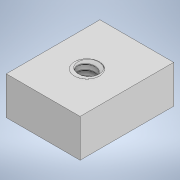
# Autodesk Inventor part: Part1
Saved by Autodesk Inventor 2020.2 (Build 242310000, 310)
## iProperties
Created: 2020-04-14
Part Number: Part1
Material: Generic
Document SubType Name: Modeling
Designer: robst
Density: 1 g/cm^3
Appearance: Default
Author: robst
Autodesk Inventor part; units mm, degrees
ref_plane "YZ Plane" through (0, 0, 0) normal (1, 0, 0) x (0, 1, 0)
ref_plane "XZ Plane" through (0, 0, 0) normal (0, 1, 0) x (-1, 0, 0)
ref_plane "XY Plane" through (0, 0, 0) normal (0, 0, 1) x (1, 0, 0)
sketch "Sketch1" plane through (0, 0, 0) normal (0, 0, 1) x (1, 0, 0)
  line L0 (-11.3242, -3.9027) -> (8.701, -3.9027)
  line L1 (8.701, -3.9027) -> (8.701, 6.3978)
  line L2 (8.701, 6.3978) -> (-11.3242, 6.3978)
  line L3 (-11.3242, 6.3978) -> (-11.3242, -3.9027)
  point P0 (0, 0)
  constraints: 8 end point, 2 parallel, 1 horizontal, 1 perpendicular
extrude "Extrusion1" add sketch "Sketch1" along normal blind 25.4
sketch "Sketch2" plane through (-11.3242, 6.3978, 0) normal (0, 1, 0) x (1, 0, 0)
  point P0 (11.3242, 0)
  point P1 (9.7887, -13.3075)
hole "Hole1" at (-1.5355, 6.3978, 13.3075) direction (0, -1, 0) diameter 6.7564 end through all clearance for "Flat Head Machine Screw (82)" size "1/4" standard "Ansi Unified Screw Threads"
thread "Thread1" size "5/16-18 UNC" class "2B" standard "ANSI Unified Screw Threads" full length
sketch "Sketch4" plane through (-1.5355, 6.3978, 13.3075) normal (1, 0, 0) x (0, 0, 1)
  line L0 (3.3782, 0) -> (3.3782, 10.3005)
  line L1 (3.3782, 10.3005) -> (2.3319, 10.3005)
  line L2 (2.3319, 10.3005) -> (2.3319, 0)
  line L3 (2.3319, 0) -> (3.3782, 0)
  line L4 (0, -3.9066) -> (0, 12.6684) projected
  constraints: 8 end point
revolve "Revolution1" add sketch "Sketch4" angle 360 about axis through (-1.5355, 6.3978, 13.3075) along (0, -1, 0) separate body
sketch "Sketch3" plane through (-1.5355, 6.3978, 16.6857) normal (-1, 0, 0) x (0, -1, 0)
  line L0 (-0.8233, -0.0715) -> (-0.7057, -0.0715) construction
  line L1 (0.1175, -0.9751) -> (-0.0001, -1.201) construction
  line L2 (-1.4112, -1.201) -> (-1.5288, -0.9751) construction
  line L3 (-0.5881, -0.0715) -> (-0.7057, 0.1544) construction
  line L4 (-0.7057, 0.1544) -> (-0.8233, -0.0715) construction
  line L5 (-1.4112, -1.201) -> (-1.2936, -0.9751) construction
  line L6 (-0.5881, -0.0715) -> (-0.1177, -0.9751)
  line L7 (-1.5288, -0.9751) -> (-1.2936, -0.9751) construction
  arc A0 (-1.5288, -0.9751) -> (-1.4112, -1.0465) centre (-1.4112, -0.9139) ccw construction
  line L8 (0.1175, -0.9751) -> (-0.1177, -0.9751) construction
  line L9 (-1.4112, -1.201) -> (-1.4112, -0.9751) construction
  line L10 (-0.0001, -1.201) -> (-0.0001, -0.9751) construction
  line L11 (-0.7057, 0.1544) -> (-0.7057, -0.0002) construction
  line L12 (-1.4112, -1.0465) -> (-0.0001, -1.0465)
  arc A1 (-1.4112, -1.0465) -> (-1.2936, -0.9751) centre (-1.4112, -0.9139) ccw
  line L13 (-0.1177, -0.9751) -> (-0.0001, -1.201) construction
  line L14 (-1.2936, -0.9751) -> (-0.8233, -0.0715)
  line L15 (-0.0001, -0.0002) -> (-0.0001, 0.0177)
  line L16 (-0.0001, 0.0177) -> (-0.0001, -0.0002)
  line L17 (-0.0001, -0.0002) -> (0.0334, -0.0002)
  arc A2 (-0.1177, -0.9751) -> (-0.0001, -1.0465) centre (-0.0001, -0.9139) ccw
  arc A3 (-0.0001, -1.0465) -> (0.1175, -0.9751) centre (-0.0001, -0.9139) ccw construction
  arc A4 (-0.7057, -0.0002) -> (-0.8233, -0.0715) centre (-0.7057, -0.1327) ccw
  arc A5 (-0.5881, -0.0715) -> (-0.7057, -0.0002) centre (-0.7057, -0.1327) ccw
  line L18 (-0.7057, -0.0002) -> (-0.7057, -0.0715) construction
  line L19 (-0.7057, -0.0715) -> (-0.5881, -0.0715) construction
  dimension "d11" = 55
  dimension "d12" = 0.2259
  dimension "d13" = 0.2259
  dimension "Sketch3_ThreadOffset" = 0
  dimension "Sketch3_MajorRadius" = 1.0463
  dimension "d16" = 1.4111
  dimension "Sketch3_MinorRadius" = 0
  constraints: 40 end point, 12 point on circle, 10 parallel, 8 tangent, 6 centre point, 6 collinear, 2 midpoint, 2 point on line, 1 horizontal, 1 perpendicular, 3 other
  measures "d11" angle of L6 L14
  measures "d12" distance of L3.end L0.end
  measures "d13" distance of L1.end L10.end
  measures "Sketch3_ThreadOffset" distance between parallel lines of L15 L10
  measures "Sketch3_MajorRadius" distance from line of L12 L15.start
  measures "d16" distance from line of L1.end L9
  measures "Sketch3_MinorRadius" distance edge to line of A5 L17
coil "Coil1" sketch "Sketch3" operation cut axis through (-1.5355, 6.3978, 13.3075) along (0, -1, 0) pitch 1.4125 turns 9.29028 hand right bodies 2
equation "\"d11\" = d18"
equation "\"d12\" = 0.160083 * Sketch3_Pitch"
equation "\"d13\" = 0.160083 * Sketch3_Pitch"
equation "\"d16\" = Sketch3_Pitch"
equation "\"d18\" = 55deg"
equation "\"Sketch3_Pitch\" = 1.41111"
body "Solid1"
body "Solid2"
